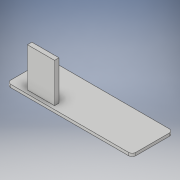
# Autodesk Inventor part: Platine
Saved by Autodesk Inventor 2019 (Build 230136000, 136)
## iProperties
Created: 2020-03-27
Part Number: Platine
Material: Generic
Document SubType Name: Modeling
Designer: Erle
Density: 1 g/cm^3
Appearance: Default
Author: Erle
Autodesk Inventor part; units mm, degrees
ref_plane "YZ Plane" through (0, 0, 0) normal (1, 0, 0) x (0, 1, 0)
ref_plane "XZ Plane" through (0, 0, 0) normal (0, 1, 0) x (-1, 0, 0)
ref_plane "XY Plane" through (0, 0, 0) normal (0, 0, 1) x (1, 0, 0)
sketch "Sketch1" plane through (0, 0, 0) normal (0, 1, 0) x (-1, 0, 0)
  line L0 (35.089, 11.43) -> (-35.089, 11.43)
  line L1 (-35.089, 11.43) -> (-35.089, -11.43)
  line L2 (-35.089, -11.43) -> (35.089, -11.43)
  line L3 (35.089, -11.43) -> (35.089, 11.43)
  line L4 (35.089, 11.43) -> (-35.089, -11.43) construction
  line L5 (-35.089, 11.43) -> (35.089, -11.43) construction
  point P0 (0, 0)
  dimension "d0" = 70.178
  dimension "d1" = 22.86
  constraints: 12 end point, 2 midpoint, 2 parallel, 1 horizontal, 1 perpendicular
  measures "d0" distance of L2.end L1.end
  measures "d1" distance between parallel lines of L0 L2
extrude "Extrusion1" add sketch "Sketch1" along normal blind 1.6
fillet "Fillet1" radius 2 4 edges at (-35.089, 0.8, -11.43) (-35.089, 0.8, 11.43) (35.089, 0.8, 11.43) (35.089, 0.8, -11.43)
sketch "Sketch7" plane through (0, 0, 0) normal (0, -1, 0) x (1, 0, 0)
  line L0 (-34.239, 0.97) -> (-27.939, 0.97)
  line L1 (-27.939, 0.97) -> (-27.939, -7.03)
  line L2 (-27.939, -7.03) -> (-34.239, -7.03)
  line L3 (-34.239, -7.03) -> (-34.239, 0.97)
  line L4 (-27.239, 0.97) -> (-20.939, 0.97)
  line L5 (-20.939, 0.97) -> (-20.939, -7.03)
  line L6 (-20.939, -7.03) -> (-27.239, -7.03)
  line L7 (-27.239, -7.03) -> (-27.239, 0.97)
  line L8 (-20.239, 0.97) -> (-13.939, 0.97)
  line L9 (-13.939, 0.97) -> (-13.939, -7.03)
  line L10 (-13.939, -7.03) -> (-20.239, -7.03)
  line L11 (-20.239, -7.03) -> (-20.239, 0.97)
  line L12 (-13.239, 0.97) -> (-6.939, 0.97)
  line L13 (-6.939, 0.97) -> (-6.939, -7.03)
  line L14 (-6.939, -7.03) -> (-13.239, -7.03)
  line L15 (-13.239, -7.03) -> (-13.239, 0.97)
  line L16 (33.089, -11.43) -> (-33.089, -11.43) projected
  line L17 (-35.089, -9.43) -> (-35.089, 9.43) projected
  point P0 (0, 0)
  point P1 (-31.089, 0.97)
  point P2 (-24.089, 0.97)
  point P3 (-17.089, 0.97)
  point P4 (-10.089, 0.97)
  point P5 (-34.239, -3.03)
  dimension "d48" = 8
  dimension "d49" = 6.3
  dimension "d50" = 6.3
  dimension "d51" = 6.3
  dimension "d52" = 6.3
  dimension "d53" = 7
  dimension "d54" = 7
  dimension "d55" = 7
  dimension "d56" = 8.4
  dimension "d85" = 4
  constraints: 32 end point, 8 parallel, 6 point on line, 5 midpoint, 4 horizontal, 4 perpendicular
  measures "d48" distance of L2.end L0.start
  measures "d49" distance of L0.start L0.end
  measures "d50" distance of L4.start L4.end
  measures "d51" distance of L8.start L8.end
  measures "d52" distance of L12.start L12.end
  measures "d53" distance of point (-24.089, 0.97) point (-31.089, 0.97)
  measures "d54" distance of point (-24.089, 0.97) point (-17.089, 0.97)
  measures "d55" distance of point (-10.089, 0.97) point (-17.089, 0.97)
  measures "d56" distance from line of L16 point (-34.239, -3.03)
  measures "d85" distance from line of L17 point (-31.089, 0.97)
extrude "Extrusion6" add sketch "Sketch7" along normal blind 2.6
sketch "Sketch8" plane through (0, -2.6, 0) normal (0, -1, 0) x (1, 0, 0)
  circle A0 centre (-31.089, -3.03) radius 1.5
  line L0 (-27.939, 0.97) -> (-34.239, 0.97) projected
  line L1 (-34.239, 0.97) -> (-34.239, -7.03) projected
  circle A1 centre (-24.089, -3.03) radius 1.5
  circle A2 centre (-17.089, -3.03) radius 1.5
  circle A3 centre (-10.089, -3.03) radius 1.5
  point P0 (0, 0)
  point P1 (-31.089, 0.97)
  point P2 (-34.239, -3.03)
  dimension "d60" = 3
  dimension "d63" = 7
  constraints: 4 centre point, 2 midpoint, 1 horizontal, 1 horizontal alignment, 1 vertical alignment, 6 other
  measures "d60" diameter of A0
  measures "d63" distance of A0.centre A1.centre
extrude "Extrusion7" add sketch "Sketch8" along normal blind 1.7
fillet "Fillet2" radius 0.5 4 edges at (-32.589, -2.6, -3.03) (-25.589, -2.6, -3.03) (-18.589, -2.6, -3.03) (-11.589, -2.6, -3.03)
sketch "Sketch9" plane through (0, 0, 0) normal (0, -1, 0) x (1, 0, 0)
  line L0 (25.289, 8.93) -> (29.089, 8.93)
  line L1 (29.089, 8.93) -> (29.089, 5.83)
  line L2 (29.089, 5.83) -> (25.289, 5.83)
  line L3 (25.289, 5.83) -> (25.289, 8.93)
  line L4 (25.289, 0.83) -> (29.089, 0.83)
  line L5 (29.089, 0.83) -> (29.089, 3.93)
  line L6 (29.089, 3.93) -> (25.289, 3.93)
  line L7 (25.289, 3.93) -> (25.289, 0.83)
  line L8 (-33.089, 11.43) -> (33.089, 11.43) projected
  line L9 (35.089, 9.43) -> (35.089, -9.43) projected
  point P0 (0, 0)
  dimension "d71" = 3.8
  dimension "d72" = 3.1
  dimension "d73" = 3.1
  dimension "d74" = 1.9
  dimension "d75" = 2.5
  dimension "d76" = 6
  constraints: 16 end point, 4 parallel, 2 horizontal, 2 perpendicular, 2 vertical alignment
  measures "d71" distance of L0.start L0.end
  measures "d72" distance of L0.end L1.end
  measures "d73" distance of L4.end L5.end
  measures "d74" distance between parallel lines of L6 L2
  measures "d75" distance between parallel lines of L8 L0
  measures "d76" distance between parallel lines of L9 L1
extrude "Extrusion8" add sketch "Sketch9" along normal blind 2
sketch "Sketch10" plane through (0, 1.6, 0) normal (0, 1, 0) x (1, 0, 0)
  line L0 (-25.589, -9.505) -> (-10.389, -9.505)
  line L1 (-10.389, -9.505) -> (-10.389, -7.005)
  line L2 (-10.389, -7.005) -> (-25.589, -7.005)
  line L3 (-25.589, -7.005) -> (-25.589, -9.505)
  line L4 (-33.089, -11.43) -> (33.089, -11.43) projected
  line L5 (-35.089, 9.43) -> (-35.089, -9.43) projected
  point P0 (0, 0)
  point P1 (-25.589, -8.255)
  dimension "d79" = 3.175
  dimension "d80" = 2.5
  dimension "d81" = 15.2
  dimension "d82" = 9.5
  constraints: 8 end point, 2 parallel, 1 horizontal, 1 midpoint, 1 perpendicular
  measures "d79" distance from line of L4 point (-25.589, -8.255)
  measures "d80" distance of L2.end L0.start
  measures "d81" distance of L1.end L2.end
  measures "d82" distance between parallel lines of L5 L3
extrude "Extrusion9" add sketch "Sketch10" along normal blind 22
body "Solid1"
